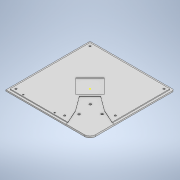
# Autodesk Inventor part: Box_Walls_2
Saved by Autodesk Inventor 2022 (Build 260153000, 153)
## iProperties
Created: 2023-02-27
Part Number: Box_Walls_2
Material: Generic
Document SubType Name: Modeling
Designer: zarek
Density: 1 g/cm^3
Appearance: Default
Author: zarek
Autodesk Inventor part; units mm, degrees
ref_plane "YZ Plane" through (0, 0, 0) normal (1, 0, 0) x (0, 1, 0)
ref_plane "XZ Plane" through (0, 0, 0) normal (0, 1, 0) x (-1, 0, 0)
sketch "Sketch1" plane through (0, 0, 0) normal (0, 1, 0) x (-1, 0, 0)
  line L0 (101.6, -101.6) -> (-101.6, -101.6)
  line L1 (-101.6, -101.6) -> (-101.6, 101.6)
  line L2 (-101.6, 101.6) -> (101.6, 101.6)
  line L3 (101.6, 101.6) -> (101.6, -101.6)
  line L4 (96.6, -96.6) -> (-96.6, -96.6)
  line L5 (-96.6, -96.6) -> (-96.6, 96.6)
  line L6 (-96.6, 96.6) -> (96.6, 96.6)
  line L7 (96.6, 96.6) -> (96.6, -96.6)
  line L8 (101.6, 101.6) -> (-40.4, 101.6)
  circle A0 centre (0, 0) radius 88.9
  circle A1 centre (0, 0) radius 109.337642
  line L9 (-40.4, 101.6) -> (-101.6, 40.4)
  line L10 (-45.4, 101.6) -> (-101.6, 45.4)
  line L11 (96.6, 96.6) -> (96.6, 101.6)
  line L12 (-45.4, 101.6) -> (-35.4, 101.6)
  line L13 (-35.4, 101.6) -> (-35.4, 96.6)
  line L14 (-35.4, 96.6) -> (-45.4, 96.6)
  line L15 (-45.4, 96.6) -> (-45.4, 101.6)
  line L16 (-45.4, 101.6) -> (-43.114, 101.6)
  line L17 (-43.114, 101.6) -> (-43.114, 96.6)
  line L18 (-43.114, 96.6) -> (-45.4, 96.6)
  line L19 (-45.4, 96.6) -> (-45.4, 101.6)
  line L20 (-96.6, 45.4) -> (-101.6, 45.4)
  line L21 (-101.6, 45.4) -> (-101.6, 43.114)
  line L22 (-101.6, 43.114) -> (-96.6, 43.114)
  line L23 (-96.6, 43.114) -> (-96.6, 45.4)
  point P0 (96.6, 51.216794)
  point P1 (101.6, 40.4)
  point P2 (101.6, -40.4)
  point P3 (96.6, -51.216794)
  point P4 (-96.6, 45.4)
  point P5 (-45.4, 96.6)
  dimension "d0" = 203.2
  dimension "d1" = 203.2
  dimension "d2" = 101.6
  dimension "d3" = 101.6
  dimension "d4" = 5
  dimension "d5" = 5
  dimension "d6" = 5
  dimension "d7" = 5
  dimension "d10" = 142
  dimension "d12" = 61.2
  dimension "d14" = 177.8
  dimension "d15" = 5
  dimension "d16" = 5
  dimension "d17" = 10
  dimension "d86" = 2.286
  dimension "d87" = 2.286
  constraints: 48 end point, 11 parallel, 10 point on line, 6 perpendicular, 5 horizontal, 2 centre point, 2 coincident, 2 point on circle
  measures "d0" distance between parallel lines of L2 L0
  measures "d1" distance between parallel lines of L1 L3
  measures "d2" distance from line of L0 point (0, 0)
  measures "d3" distance from line of L1 point (0, 0)
  measures "d4" distance between parallel lines of L4 L0
  measures "d5" distance between parallel lines of L1 L5
  measures "d6" distance between parallel lines of L2 L6
  measures "d7" distance between parallel lines of L3 L7
  measures "d10" distance of L2.end L8.end
  measures "d12" distance from line of L1 L8.end
  measures "d14" diameter of A0
  measures "d15" distance of L10.end L9.end
  measures "d16" distance of L10.start L8.end
  measures "d17" distance of L13.end L14.end
  measures "d86" distance of L17.end L18.end
  measures "d87" distance of L21.end L20.end
extrude "Extrusion1" add sketch "Sketch1" along normal blind 5 contours L0 A1 L4 L7 L3 | L0 A1 L4 | A1 L7 L3 | L0 L1 A1 L5 L4 | A1 L7 L4 | L4 A1 L5 L9 L6 L7 | A1 L7 L11 L2 L3 | L4 L5 A1 | A1 L6 L7 | L1 L9 L22 L5 A1 | L11 L6 A1 L2 | L6 L13 L2 A1 | L1 L22 A1 | A1 L22 L9 | L22 L9 L5 | L6 L17 L9 L2 L13 | L1 L20 A1 L22 | A1 L20 L9 L22 | L20 A1 L10 L5 | L5 L10 L6 L9 | A1 L17 L2 | L9 L17 A1 | L6 L9 L17 | L1 L2 L10 A1 L6 L5 | L10 A1 L20 | L10 A1 L5 | L5 A1 L6 L10 | L15 A1 L17 L9 | L6 L10 A1 L15 | L17 A1 L15 L2 | L5 L6 A1 | L6 A1 L10 | A1 L10 L15 | A0
sketch "Sketch3" plane through (0, 5, 0) normal (0, 1, 0) x (1, 0, 0)
  circle A0 centre (0, 0) radius 88.9
  line L0 (-101.6, 101.6) -> (-101.6, -101.6)
  line L1 (-101.6, -101.6) -> (101.6, -101.6)
  line L2 (-101.6, 101.6) -> (101.6, 101.6)
  line L3 (101.6, 101.6) -> (101.6, -101.6)
  line L4 (101.6, -101.6) -> (-101.6, -101.6)
  line L5 (-101.6, -101.6) -> (-101.6, 101.6)
  line L6 (-96.6, 96.6) -> (96.6, 96.6)
  line L7 (96.6, 96.6) -> (96.6, -96.6)
  line L8 (96.6, -96.6) -> (-96.6, -96.6)
  line L9 (-96.6, -96.6) -> (-96.6, 96.6)
  line L10 (-101.6, -101.6) -> (40.4, -101.6)
  circle A1 centre (0, 0) radius 109.337642
  line L11 (40.4, -101.6) -> (101.6, -40.4)
  line L12 (101.6, -101.6) -> (101.6, 101.6)
  line L13 (45.4038, -101.6) -> (101.6, -45.4038)
  line L14 (96.6, -45.4) -> (101.6, -45.4038)
  line L15 (45.4, -96.6) -> (45.4038, -101.6)
  line L16 (96.6, -45.4) -> (101.6, -45.4)
  line L17 (101.6, -45.4) -> (101.6, -43.114)
  line L18 (101.6, -43.114) -> (96.6, -43.114)
  line L19 (96.6, -43.114) -> (96.6, -45.4)
  line L20 (45.4038, -101.6) -> (43.1178, -101.6)
  line L21 (43.1178, -101.6) -> (43.1178, -96.6)
  line L22 (43.1178, -96.6) -> (45.4038, -96.6)
  line L23 (45.4038, -96.6) -> (45.4038, -101.6)
  point P0 (45.4038, -101.6)
  point P1 (50.4038, -96.6)
  point P2 (96.6, -50.4038)
  dimension "d28" = 177.8
  dimension "d29" = 5
  dimension "d30" = 5
  dimension "d31" = 5
  dimension "d32" = 5
  dimension "d33" = 142
  dimension "d76" = 5.0038
  dimension "d77" = 5.0038
  dimension "d88" = 2.286
  dimension "d89" = 2.286
  constraints: 42 end point, 10 point on line, 9 parallel, 4 horizontal, 4 perpendicular, 2 centre point, 2 coincident, 2 point on circle
  measures "d28" diameter of A0
  measures "d29" distance between parallel lines of L3 L7
  measures "d30" distance between parallel lines of L6 L2
  measures "d31" distance between parallel lines of L0 L9
  measures "d32" distance between parallel lines of L1 L8
  measures "d33" distance of L4.end L10.end
  measures "d76" distance of L13.end L11.end
  measures "d77" distance of L13.start L10.end
  measures "d88" distance of L17.end L16.end
  measures "d89" distance of L21.end L22.end
extrude "Extrusion3" cut sketch "Sketch3" against normal blind 2 contours L2 A1 L6 L9 L0 | A1 L9 L0 | L2 A1 L6 | A1 L9 L8 L1 L0 | L2 L3 A1 L7 L6 | A1 L8 L21 L11 L1 | L3 L11 L18 L7 A1 | A1 L21 L1 | L11 L21 A1 | L3 L18 A1 | A1 L18 L11
sketch "Sketch4" plane through (0, 5, 0) normal (0, 1, 0) x (1, 0, 0)
  line L0 (101.6, 101.6) -> (-101.6, 101.6)
  line L1 (-101.6, 101.6) -> (-101.6, -101.6)
  line L2 (-101.6, -101.6) -> (101.6, -101.6)
  line L3 (101.6, -101.6) -> (101.6, 101.6)
  circle A0 centre (0, 0) radius 2.5
  line L4 (11.331386, 2.138998) -> (-2.138998, -11.331386)
  line L5 (0, 0) -> (-5.656854, 5.656854)
  line L6 (-5.656854, -14.849242) -> (-26.162951, 5.656855)
  line L7 (-5.656854, 26.162952) -> (14.849242, 5.656855)
  circle A1 centre (-5.656854, 5.656854) radius 14
  line L8 (-26.162951, 5.656855) -> (-5.656854, 26.162952)
  line L9 (14.849242, 5.656855) -> (-5.656854, -14.849242)
  line L10 (-40.305087, 5.656855) -> (-5.656854, 40.305087)
  line L11 (-5.656854, 40.305087) -> (28.991378, 5.656855)
  line L12 (28.991378, 5.656855) -> (-5.656854, -28.991377)
  line L13 (-5.656854, -28.991377) -> (-40.305087, 5.656855)
  line L14 (-22.645095, 9.174711) -> (-9.174711, 22.645095)
  line L15 (-9.174711, 22.645095) -> (-12.766813, 26.237197)
  line L16 (-12.766813, 26.237197) -> (-26.237197, 12.766813)
  line L17 (-26.237197, 12.766813) -> (-22.645095, 9.174711)
  point P0 (9.525, 22.5)
  point P1 (-9.525, -6.5)
  dimension "d37" = 203.2
  dimension "d38" = 203.2
  dimension "d39" = 8
  dimension "d40" = 28
  dimension "d41" = 29
  dimension "d42" = 29
  dimension "d43" = 14.5
  dimension "d44" = 10
  dimension "d45" = 10
  dimension "d46" = 10
  dimension "d47" = 10
  dimension "d48" = 5.08
  dimension "d49" = 9.525
  dimension "d50" = 9.525
  dimension "d55" = 101.6
  dimension "d56" = 101.6
  constraints: 36 end point, 8 parallel, 4 perpendicular, 2 centre point, 2 coincident, 2 point on line, 1 horizontal
  measures "d37" distance between parallel lines of L2 L0
  measures "d38" distance between parallel lines of L1 L3
  measures "d39" distance of L5.start L5.end
  measures "d40" diameter of A1
  measures "d41" distance between parallel lines of L9 L8
  measures "d42" distance between parallel lines of L7 L6
  measures "d43" distance from line of A1.centre L8
  measures "d44" distance between parallel lines of L11 L7
  measures "d45" distance between parallel lines of L8 L10
  measures "d46" distance between parallel lines of L13 L6
  measures "d47" distance between parallel lines of L12 L9
  measures "d48" distance between parallel lines of L14 L16
  measures "d49" distance from line of A1.centre L15
  measures "d50" distance from line of L5.end L17
  measures "d55" distance from line of point (0, 0) L1
  measures "d56" distance from line of L0 point (0, 0)
extrude "Extrusion4" cut sketch "Sketch4" against normal blind 1 contours A0 | L4 L9 L6 L8 L7 | L8 L17 L16 L15 | A1 | L10 L11 L12 L13
sketch "Sketch6" plane through (0, 5, 0) normal (0, 1, 0) x (1, 0, 0)
  line L0 (45.4038, -101.6) -> (0, 0)
  line L1 (50.4038, -96.6) -> (45.4038, -101.6)
  line L2 (96.6, -43.114) -> (96.6, 96.6)
  line L3 (101.6, -101.6) -> (101.6, 101.6)
  circle A0 centre (0, 0) radius 34.925
  circle A1 centre (0, 0) radius 33.425
  line L4 (-101.6, 101.6) -> (-101.6, -101.6)
  line L5 (-101.6, -101.6) -> (40.4, -101.6)
  line L6 (-101.6, -101.6) -> (101.6, -101.6)
  line L7 (101.6, 101.6) -> (101.6, -43.114)
  line L8 (101.6, -45.4038) -> (0, 0)
  line L9 (-96.6, -96.6) -> (43.1178, -96.6)
  line L10 (96.6, -43.114) -> (96.6, 96.6)
  line L11 (43.1178, -101.6) -> (-101.6, -101.6)
  line L12 (101.6, -45.4038) -> (96.6, -50.4038)
  line L13 (45.4038, -101.6) -> (101.6, -45.4038)
  line L14 (43.1178, -101.6) -> (101.6, -101.6)
  line L15 (0, 0) -> (101.6, -50.4076)
  line L16 (50.4076, -101.6) -> (0, 0)
  line L17 (43.169361, -96.6) -> (47.926911, -96.6)
  line L18 (96.6, -43.169361) -> (96.6, -47.926911)
  line L19 (40.4, -101.6) -> (101.6, -40.4)
  point P0 (13.637413, -30.516415)
  point P1 (30.516415, -13.637413)
  point P2 (14.249414, -31.885888)
  point P3 (31.286053, -15.522194)
  point P4 (29.942343, -14.855528)
  point P5 (31.885888, -14.249414)
  point P6 (98.255522, -48.748278)
  point P7 (96.6, -47.926911)
  point P8 (47.926911, -96.6)
  point P9 (15.522194, -31.286053)
  point P10 (96.6, -45.4)
  point P11 (45.4, -96.6)
  point P12 (14.855528, -29.942343)
  point P13 (96.6, -45.4)
  point P14 (45.4, -96.6)
  point P15 (45.4, -96.6)
  point P16 (47.088956, -94.911044)
  point P17 (94.911044, -47.088956)
  point P18 (96.6, -45.4)
  point P19 (43.858319, -98.141681)
  point P20 (98.141681, -43.858319)
  point P21 (45.4, -96.6)
  point P22 (96.6, -45.4)
  dimension "d71" = 69.85
  dimension "d72" = 66.85
  dimension "d75" = 142
  dimension "d78" = 5.0038
  dimension "d82" = 5.0038
  constraints: 18 end point, 11 point on line, 2 centre point, 2 coincident, 1 collinear, 1 perpendicular
  measures "d71" diameter of A0
  measures "d72" diameter of A1
  measures "d75" distance of L4.end L5.end
  measures "d78" distance of L0.start L5.end
  measures "d82" distance of L8.start L19.end
extrude "Extrusion6" cut sketch "Sketch6" against normal blind 1 contours L0 A0 L16 L19 L17 | L0 A1 L16 A0 | L16 A1 L15 A0 | L15 A0 L8 L18 L19 | A0 L15 A1 L8
fillet "Fillet3" radius 12.7 1 edges at (101.6, 2.5, 101.6)
sketch "Sketch9" plane through (0, 4, 0) normal (0, 1, 0) x (1, 0, 0)
  point P0 (0, 0)
sketch "Sketch10" plane through (0, 5, 0) normal (0, 1, 0) x (1, 0, 0)
  point P0 (0, 0)
ref_plane "Work Plane1" through (24.695704, 5, 24.695704) normal (0.7071068, 0, 0.7071068) x (0.7071068, 0, -0.7071068)
sketch "Sketch15" plane through (0, 5, 0) normal (0, 1, 0) x (1, 0, 0)
  line L0 (43.169361, -96.6) -> (13.637413, -30.516415)
  line L1 (28.403387, -63.558207) -> (-0.656854, -23.991377)
  line L2 (28.991378, 5.656855) -> (-5.656854, -28.991377)
  line L3 (30.516415, -13.637413) -> (96.6, -43.169361)
  line L4 (-5.656854, 40.305087) -> (28.991378, 5.656855)
  line L5 (63.558207, -28.403387) -> (23.991378, 0.656855)
  line L6 (2.337401, -28.06819) -> (28.068191, -2.3374)
  arc A0 (13.637413, -30.516415) -> (30.516415, -13.637413) centre (0, 0) ccw
  line L7 (28.403387, -63.558207) -> (13.637413, -30.516415)
  line L8 (63.558207, -28.403387) -> (30.516415, -13.637413)
  arc A1 (13.637413, -30.516415) -> (30.516415, -13.637413) centre (0, 0) ccw
  line L9 (28.619467, -64.395349) -> (1.630294, -28.775297)
  line L10 (1.630294, -28.775297) -> (2.337401, -28.06819)
  dimension "d138" = 5
  dimension "d139" = 5
  dimension "d140" = 5
  dimension "d168" = 1
  constraints: 14 end point, 4 point on line, 3 point on circle, 2 midpoint, 1 centre point, 1 collinear, 1 concentric, 1 parallel
  measures "d138" horizontal distance of L2.end L1.end
  measures "d139" horizontal distance of L2.start L5.end
  measures "d140" distance between parallel lines of L6 L2
  measures "d168" distance of L6.start L9.end
extrude "Extrusion11" cut sketch "Sketch15" against normal blind 1 contours L1 L6 L5 L3 A0 L0
sketch "Sketch16" plane through (0, 4, 0) normal (0, 1, 0) x (1, 0, 0)
  line L0 (2.337401, -28.06819) -> (28.068191, -2.3374)
  line L1 (9.408468, -20.997123) -> (12.944002, -24.532656)
  line L2 (12.944002, -24.532656) -> (24.532657, -12.944002)
  line L3 (24.532657, -12.944002) -> (20.997123, -9.408468)
  line L4 (12.944002, -24.532656) -> (24.532657, -12.944002)
  line L5 (24.532657, -12.944002) -> (28.559218, -16.970562)
  line L6 (28.559218, -16.970562) -> (16.970563, -28.559217)
  line L7 (16.970563, -28.559217) -> (12.944002, -24.532656)
  line L8 (12.944002, -24.532656) -> (5.331655, -32.145003)
  line L9 (28.403387, -63.558207) -> (2.337401, -28.06819)
  line L10 (24.532657, -12.944002) -> (32.145004, -5.331655)
  line L11 (28.068191, -2.3374) -> (63.558207, -28.403387)
  point P0 (0, 0)
  dimension "d144" = 10
  dimension "d145" = 10
  dimension "d146" = 5
  dimension "d152" = 0
  dimension "d153" = 0
  constraints: 18 end point, 6 perpendicular, 6 point on line
  measures "d144" distance of L0.start L1.start
  measures "d145" distance of L0.end L3.end
  measures "d146" distance between parallel lines of L0 L2
  measures "d152" distance between parallel lines of L7 L1
  measures "d153" distance between parallel lines of L5 L3
extrude "Extrusion12" cut sketch "Sketch16" along normal up to surface (1 mm away)
sketch "Sketch20" plane through (0, 5, 0) normal (0, 1, 0) x (1, 0, 0)
  line L0 (47.088956, -94.911044) -> (45.4, -96.6)
  line L1 (47.088956, -94.911044) -> (94.937604, -47.062396)
  line L2 (94.164915, -47.835085) -> (33.507042, -17.740422)
  line L3 (94.911044, -47.088956) -> (31.286053, -15.522194)
  line L4 (15.522194, -31.286053) -> (47.088956, -94.911044)
  line L5 (17.526471, -33.075809) -> (47.835085, -94.164915)
  arc A0 (15.522194, -31.286053) -> (31.286053, -15.522194) centre (0, 0) ccw
  line L6 (33.507042, -17.740422) -> (31.719266, -16.853439)
  line L7 (17.526471, -33.075809) -> (16.753056, -31.516938)
  arc A1 (16.753056, -31.516938) -> (31.719266, -16.853439) centre (3.790359, -3.317307) ccw
  dimension "d169" = 1
  dimension "d172" = 1
  constraints: 10 end point, 2 point on circle, 2 point on line, 1 centre point, 1 collinear, 1 parallel
  measures "d169" distance between parallel lines of L2 L3
  measures "d172" distance between parallel lines of L5 L4
extrude "Extrusion13" cut sketch "Sketch20" against normal blind 1 contours L4 A0 L3 L1 L2 L6 A1 L7 L5
sketch "Sketch21" plane through (0, 5, 0) normal (0, 1, 0) x (1, 0, 0)
  line L0 (31.719266, -10.124493) -> (13.677789, -27.994866)
  line L1 (47.835085, -94.164915) -> (45.4, -96.6)
  line L2 (13.677789, -27.994866) -> (47.835085, -94.164915)
  line L3 (47.835085, -94.164915) -> (43.1178, -96.6)
  line L4 (43.1178, -96.6) -> (43.1178, -101.6)
  line L5 (43.1178, -96.6) -> (43.1178, -101.6)
  line L6 (43.1178, -101.6) -> (100.933808, -101.6)
  line L7 (100.933808, -101.6) -> (101.6, -101.6)
  line L8 (101.6, 101.6) -> (101.6, -43.114)
  line L9 (101.6, -43.114) -> (101.6, -101.6)
  line L10 (101.6, -88.9) -> (101.6, 101.6)
  line L11 (101.6, -43.114) -> (96.6, -43.114)
  line L12 (96.6, -43.114) -> (91.337275, -46.432186)
  line L13 (94.164915, -47.835085) -> (31.719266, -16.853439)
  line L14 (91.337275, -46.432186) -> (27.19303, -14.607802)
  constraints: 20 end point, 3 collinear, 3 point on line, 2 perpendicular, 1 horizontal
extrude "Extrusion14" cut sketch "Sketch21" against normal blind 1
sketch "Sketch22" plane through (0, 5, 0) normal (0, 1, 0) x (1, 0, 0)
  point P0 (0, 0)
sketch "Sketch25" plane through (0, 5, 0) normal (0, 1, 0) x (1, 0, 0)
  line L0 (-96.6, 96.6) -> (-96.6, -96.6)
  line L1 (96.6, 96.6) -> (-96.6, 96.6)
  line L2 (-96.6, 96.6) -> (96.6, 96.6)
  line L3 (96.6, -45.4) -> (45.4, -96.6)
  line L4 (96.6, 96.6) -> (96.6, -45.4)
  line L5 (96.6, -45.4) -> (45.4, -96.6)
  line L6 (45.4, -96.6) -> (-96.6, -96.6)
  line L7 (-96.6, -96.6) -> (-96.6, 96.6)
  line L8 (-96.6, 96.6) -> (-89.528932, 89.528932)
  circle A0 centre (-89.528932, 89.528932) radius 5
  circle A1 centre (-89.528932, 89.528932) radius 1.5
  line L9 (-89.528932, 84.528932) -> (-96.6, 84.528932)
  line L10 (-89.528932, 89.528932) -> (-89.528932, 84.528932)
  line L11 (-89.528932, 89.528932) -> (-84.528932, 89.528932)
  line L12 (-84.528932, 96.6) -> (-84.528932, 89.528932)
  line L13 (-96.6, -96.6) -> (-89.528932, -89.528932)
  line L14 (-96.6, -96.6) -> (-86.6, -96.6) construction
  circle A2 centre (-89.528932, -89.528932) radius 5
  circle A3 centre (-89.528932, -89.528932) radius 1.75
  line L15 (-89.528932, -89.528932) -> (-84.528932, -89.528932)
  line L16 (-84.528932, -96.6) -> (-84.528932, -89.528932)
  line L17 (-89.528932, -89.528932) -> (-89.528932, -84.528932)
  line L18 (-96.6, -84.528932) -> (-89.528932, -84.528932)
  line L19 (96.6, 96.6) -> (89.528932, 89.528932)
  circle A4 centre (89.528932, 89.528932) radius 5
  circle A5 centre (89.528932, 89.528932) radius 1.75
  line L20 (89.528932, 89.528932) -> (84.528932, 89.528932)
  line L21 (84.528932, 96.6) -> (84.528932, 89.528932)
  line L22 (89.528932, 89.528932) -> (89.528932, 84.528932)
  line L23 (96.6, 84.528932) -> (89.528932, 84.528932)
  line L24 (96.6, -43.114) -> (96.6, 96.6)
  line L25 (-96.6, -96.6) -> (43.1178, -96.6)
  line L26 (28.991378, 5.656855) -> (-5.656854, -28.991377)
  line L27 (25.4, -25.4) -> (101.6, -25.4)
  line L28 (101.6, -88.9) -> (101.6, 101.6)
  line L29 (25.4, -25.4) -> (25.4, -101.6)
  line L30 (43.1178, -101.6) -> (-101.6, -101.6)
  line L31 (96.6, -25.4) -> (86.6, -25.4)
  circle A6 centre (86.6, -25.4) radius 5
  circle A7 centre (86.6, -25.4) radius 1.75
  line L32 (25.4, -96.6) -> (25.4, -86.6)
  circle A8 centre (25.4, -86.6) radius 5
  circle A9 centre (25.4, -86.6) radius 1.75
  point P0 (0, 0)
  dimension "d203" = 10
  dimension "d205" = 3
  dimension "d206" = 10
  dimension "d207" = 45
  dimension "d208" = 10
  dimension "d209" = 3.5
  dimension "d210" = 10
  dimension "d211" = 10
  dimension "d212" = 3.5
  dimension "d223" = 76.2
  dimension "d224" = 76.2
  dimension "d225" = 10
  dimension "d226" = 10
  dimension "d227" = 3.5
  dimension "d228" = 10
  dimension "d229" = 10
  dimension "d230" = 3.5
  constraints: 50 end point, 14 point on line, 10 centre point, 9 coincident, 9 perpendicular, 6 point on circle, 5 horizontal, 3 parallel, 2 tangent, 1 collinear, 1 equal length, 1 vertical
  measures "d203" distance of L0.start L8.end
  measures "d205" diameter of A1
  measures "d206" distance of L6.end L13.end
  measures "d207" angle of L14 L13
  measures "d208" diameter of A2
  measures "d209" diameter of A3
  measures "d210" distance of L1.start L19.end
  measures "d211" diameter of A4
  measures "d212" diameter of A5
  measures "d223" distance between parallel lines of L28 L29
  measures "d224" distance between parallel lines of L30 L27
  measures "d225" distance of L31.start L31.end
  measures "d226" diameter of A6
  measures "d227" diameter of A7
  measures "d228" distance of L32.start L32.end
  measures "d229" diameter of A8
  measures "d230" diameter of A9
hole "Hole3" at (-89.528932, 5, 89.528932) at (-89.528932, 5, -89.528932) at (89.528932, 5, -89.528932) at (25.4, 5, 86.6) at (86.6, 5, 25.4) direction (0, -1, 0) diameter 2.85 depth 12.7 tip angle 118 countersink diameter 4.445 countersink angle 82 thread size "M3.5x0.6" class "6H" standard "ANSI Metric M Profile"
sketch "Sketch26" plane through (0, 5, 0) normal (0, 1, 0) x (1, 0, 0)
  line L0 (-96.6, -92.679258) -> (-96.6, -59.679258)
  line L1 (-68.6, -92.679258) -> (-96.6, -92.679258)
  line L2 (-96.6, -96.6) -> (43.1178, -96.6)
  line L3 (-68.6, -92.679258) -> (-68.6, -96.6)
  line L4 (-68.6, -92.679258) -> (7.4, -92.679258)
  circle A0 centre (-68.6, -92.679258) radius 1.5
  circle A1 centre (7.4, -92.679258) radius 1.5
  line L5 (-101.6, -101.6) -> (-101.6, 101.6)
  point P0 (0, 0)
  dimension "d232" = 3.92074
  dimension "d234" = 76
  dimension "d235" = 3
  dimension "d236" = 3
  dimension "d244" = 33
  constraints: 8 end point, 2 centre point, 2 coincident, 2 horizontal, 1 perpendicular, 1 point on line
  measures "d232" distance between parallel lines of L2 L1
  measures "d234" distance of L1.start L4.end
  measures "d235" diameter of A0
  measures "d236" diameter of A1
  measures "d244" distance from line of L5 L1.start
hole "Hole4" at (-68.6, 5, 92.679258) at (7.4, 5, 92.679258) direction (0, -1, 0) diameter 2.85 depth 2.54 tip angle 118 countersink diameter 3.175 countersink angle 82 thread size "M3.5x0.6" class "6H" standard "ANSI Metric M Profile"
sketch "Sketch28" plane through (0, 0, 0) normal (0, -1, 0) x (1, 0, 0)
  circle A0 centre (-6.381482, -33.94934) radius 1.425
  circle A1 centre (-6.381482, -33.94934) radius 1.425
  circle A2 centre (-33.953993, -6.376829) radius 1.425
  circle A3 centre (-33.953993, -6.376829) radius 1.425
  circle A4 centre (-5.28314, 22.294025) radius 1.425
  circle A5 centre (-5.28314, 22.294025) radius 1.425
  circle A6 centre (22.289371, -5.278486) radius 1.5113
  circle A7 centre (22.289371, -5.278486) radius 1.5113
  point P0 (0, 0)
  point P1 (0, 0)
  constraints: 8 centre point, 4 coincident
fillet "Fillet5" radius 3.175 2 edges at (101.6, 1.5, -101.6) (-101.6, 1.5, -101.6)
sketch "Sketch29" plane through (0, 4, 0) normal (0, 1, 0) x (1, 0, 0)
  line L0 (96.6, -43.114) -> (96.6, 96.6)
  line L1 (0, 0) -> (18.582937, 0.245427)
  line L2 (0, 0) -> (0.183127, -13.865783)
  line L3 (0, 0) -> (31.843231, -31.01308)
  circle A0 centre (31.843231, -31.01308) radius 2.6
  line L4 (0, 0) -> (38.968155, -65.482234)
  line L5 (0, 0) -> (66.488529, -37.225201)
  circle A1 centre (66.488529, -37.225201) radius 2.6
  circle A2 centre (38.968155, -65.482234) radius 2.6
  dimension "d266" = 5.2
  dimension "d267" = 44.45
  dimension "d268" = 76.2
  dimension "d269" = 76.2
  dimension "d270" = 15
  dimension "d271" = 15
  dimension "d272" = 5.2
  dimension "d273" = 5.2
  dimension "d274" = 30
  dimension "d275" = 30
  constraints: 10 end point, 3 centre point, 3 coincident
  measures "d266" diameter of A0
  measures "d267" distance of L1.start L3.end
  measures "d268" distance of L1.start L4.end
  measures "d269" distance of L1.start L5.end
  measures "d270" angle of L3 L5
  measures "d271" angle of L4 L3
  measures "d272" diameter of A1
  measures "d273" diameter of A2
  measures "d274" angle of L2 L4
  measures "d275" angle of L1 L5
extrude "Extrusion16" cut sketch "Sketch29" against normal blind 2.2
equation "\"d1\" = d0"
equation "\"d2\" = 0.5 * d0"
equation "\"d3\" = 0.5 * d0"
body "Solid1"
